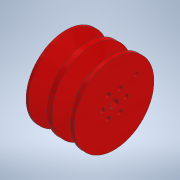
# Autodesk Inventor part: Gobilda winch pulley adapter V3
Saved by Autodesk Inventor 2022 (Build 260153000, 153)
## iProperties
Created: 2022-11-29
Part Number: Gobilda winch pulley adapter V3
Material: Generic
Document SubType Name: Modeling
Designer: matt
Density: 1 g/cm^3
Appearance: Default
Author: matt
Autodesk Inventor part; units mm, degrees
ref_plane "YZ Plane" through (0, 0, 0) normal (1, 0, 0) x (0, 1, 0)
ref_plane "XZ Plane" through (0, 0, 0) normal (0, 1, 0) x (-1, 0, 0)
ref_plane "XY Plane" through (0, 0, 0) normal (0, 0, 1) x (1, 0, 0)
sketch "Sketch2" plane through (0, 0, 0) normal (1, 0, 0) x (0, 1, 0)
  circle A0 centre (0, 0) radius 26.9875
  circle A1 centre (0, 0) radius 16.25
  circle A2 centre (-6.928203, 4) radius 1.7
  circle A3 centre (0, 8) radius 1.7
  line L0 (-9.192388, 9.192388) -> (0, 0) construction
  line L1 (-1.616581, 2.8) -> (1.616581, 2.8)
  line L2 (1.616581, 2.8) -> (3.233162, 0)
  line L3 (-3.233162, 0) -> (-1.616581, 2.8)
  line L4 (1.616581, -2.8) -> (-1.616581, -2.8)
  line L5 (3.233162, 0) -> (1.616581, -2.8)
  circle A4 centre (-6.928203, -4) radius 1.7
  line L6 (-1.616581, -2.8) -> (-3.233162, 0)
  circle A5 centre (6.928203, -4) radius 1.7
  circle A6 centre (6.928203, 4) radius 1.7
  circle A7 centre (0, -8) radius 1.7
  circle A8 centre (0, 0) radius 26
  circle A9 centre (9.845928, -14.768893) radius 1.5
  point P0 (2.343467, 17.800401)
  point P1 (0, 18.524)
  dimension "d27" = 3.4
  dimension "d28" = 8
  dimension "d29" = 360
  dimension "d30" = 13
  dimension "d31" = 5.6
  dimension "d32" = 32.5
  dimension "d33" = 52
  dimension "d34" = 3
  constraints: 14 end point, 10 centre point, 6 coincident, 1 tangent, 26 other
  measures "d27" diameter of A3
  measures "d28" distance of point (0, 0) A3.centre
  measures "d30" distance of point (0, 0) L0.start
  measures "d31" distance between parallel lines of L4 L1
  measures "d32" diameter of A1
  measures "d33" diameter of A8
  measures "d34" diameter of A9
sketch "Sketch1" plane through (0, 0, 0) normal (0, 0, 1) x (1, 0, 0)
  line L0 (1.135068, 26.966581) -> (7.280551, 16.322293)
  line L1 (23.219449, 16.322293) -> (29.364932, 26.966581)
  line L2 (12, 16.322293) -> (12, 0) construction
  line L3 (18.5, 16.322293) -> (18.5, 0) construction
  line L4 (25.5, 16.322293) -> (25.5, 0) construction
  line L5 (32, 26) -> (32, 0)
  line L6 (15.25, 25.901488) -> (15.25, 10.116581) construction
  line L7 (8.5, 14.210145) -> (8.5, 8.416581) construction
  line L8 (22, 14.210145) -> (22, 8.416581) construction
  line L9 (22, 8.416581) -> (22, 11.916581) construction
  line L10 (5, 14.210145) -> (25.5, 14.210145) construction
  line L11 (5, 16.322293) -> (7.280551, 16.322293) construction
  line L12 (7.280551, 16.322293) -> (9.316, 16.322293)
  line L13 (9.719449, 16.322293) -> (20.780551, 16.322293) construction
  line L14 (21.177933, 16.322293) -> (23.219449, 16.322293)
  line L15 (23.219449, 16.322293) -> (25.5, 16.322293) construction
  line L16 (-0.72931, 26.966581) -> (-0.72931, 20.143218)
  line L17 (-0.72931, 20.143218) -> (3.5, 13.716393)
  line L18 (0, 4.924977) -> (0, 0)
  line L19 (0, 0) -> (32, 0)
  line L20 (32, 25.901488) -> (32, 0)
  line L21 (0, 0) -> (0, 10.666581)
  line L22 (0, 10.666581) -> (3.5, 10.666581)
  line L23 (3.5, 13.716393) -> (3.5, 10.666581)
  line L24 (32, 26.966581) -> (32, 25.901488)
  line L25 (9.316, 16.322293) -> (13.428275, 26.966581)
  line L26 (21.177933, 16.322293) -> (17.035083, 26.966581)
  line L27 (29.364932, 26.966581) -> (32, 26.966581)
  line L28 (-0.72931, 26.966581) -> (1.135068, 26.966581)
  line L29 (13.428275, 26.966581) -> (17.035083, 26.966581)
  dimension "d19" = 6.5
  dimension "d20" = 3.25
  dimension "d21" = 3.5
  dimension "d22" = 3.5
  constraints: 60 end point, 11 point on line, 9 perpendicular, 1 collinear
  measures "d19" distance between parallel lines of L3 L2
  measures "d20" distance between parallel lines of L3 L6
  measures "d21" distance between parallel lines of L4 L9
  measures "d22" distance between parallel lines of L2 L7
sweep "Sweep1" add profiles "Sketch1" path "Sketch2" path curves A0
sketch "Sketch2 outline for Extrusion1" plane through (0, 0, 0) normal (1, 0, 0) x (0, 1, 0)
  circle A0 centre (0, -8) radius 1.7
  circle A1 centre (-6.928203, -4) radius 1.7
  circle A2 centre (-6.928203, 4) radius 1.7
  circle A3 centre (0, 8) radius 1.7
  line L0 (-1.616581, 2.8) -> (-3.233162, 0)
  line L1 (1.616581, 2.8) -> (-1.616581, 2.8)
  line L2 (3.233162, 0) -> (1.616581, 2.8)
  line L3 (1.616581, -2.8) -> (3.233162, 0)
  line L4 (-1.616581, -2.8) -> (1.616581, -2.8)
  line L5 (-3.233162, 0) -> (-1.616581, -2.8)
  circle A4 centre (6.928203, 4) radius 1.7
  circle A5 centre (6.928203, -4) radius 1.7
  circle A6 centre (9.845928, -14.768893) radius 1.5
extrude "Extrusion1" cut sketch "Sketch2 outline for Extrusion1" along normal through all
body "Solid1"
